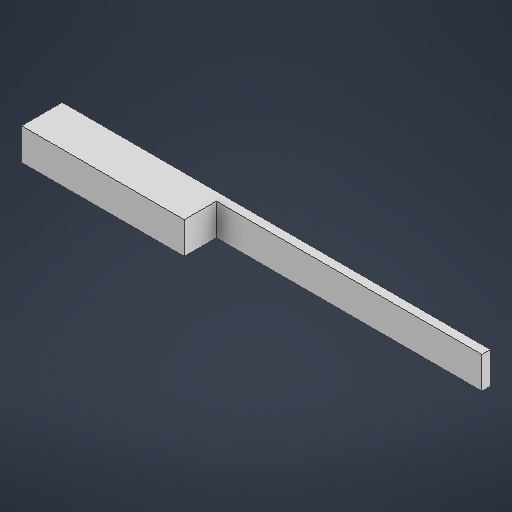
# Autodesk Inventor part: ведро 2 гол
Saved by Autodesk Inventor 2025 (Build 290162000, 162)
## iProperties
Created: 2025-01-16
Part Number: ведро 2 гол
Material: Типовые
Document SubType Name: Modeling
Designer: Phantom
Density: 1 g/cm^3
Appearance: По умолчанию
Author: Phantom
Autodesk Inventor part; units mm, degrees
ref_plane "YZ Plane" through (0, 0, 0) normal (1, 0, 0) x (0, 1, 0)
ref_plane "XZ Plane" through (0, 0, 0) normal (0, 1, 0) x (-1, 0, 0)
ref_plane "XY Plane" through (0, 0, 0) normal (0, 0, 1) x (1, 0, 0)
sketch "Эскиз1" plane through (0, 0, 0) normal (0, 0, 1) x (1, 0, 0)
  line L0 (0, 0) -> (200, 0)
  line L1 (200, 0) -> (200, 14.8438)
  line L2 (200, 14.8438) -> (0, 14.8438)
  line L3 (0, 14.8438) -> (0, 0)
  dimension "d2" = 200
  constraints: 8 end point, 2 parallel, 1 horizontal, 1 perpendicular
  measures "d2" distance of L1.end L2.end
extrude "Выдавливание1" add sketch "Эскиз1" along normal blind 4
sketch "Эскиз2" plane through (0, 0, 4) normal (0, 0, 1) x (1, 0, 0)
  line L0 (200, 14.8438) -> (0, 14.8438) projected
  line L1 (0, 0) -> (200, 0) projected
  line L2 (0, 14.8438) -> (76, 14.8438)
  line L3 (76, 14.8438) -> (76, 0)
  line L4 (76, 0) -> (0, 0)
  line L5 (0, 0) -> (0, 14.8438)
  constraints: 8 end point, 2 parallel, 1 horizontal, 1 perpendicular, 1 point on line
extrude "Выдавливание2" add sketch "Эскиз2" along normal blind 15
